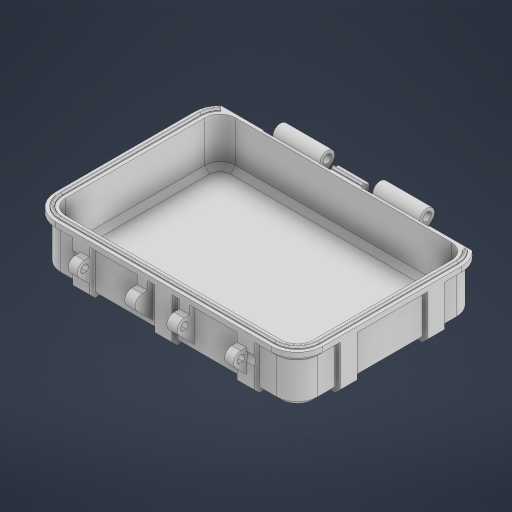
# Autodesk Inventor part: universal_box-lid
Saved by Autodesk Inventor 2024 (Build 280153000, 153)
## iProperties
Created: 2024-03-05
Part Number: universal_box-lid
Material: Všeobecné
Document SubType Name: Modeling
Designer: Simak
Density: 1 g/cm^3
Appearance: Výchozí
Author: Simak
Autodesk Inventor part; units mm, degrees
ref_plane "YZ Plane" through (0, 0, 0) normal (1, 0, 0) x (0, 1, 0)
ref_plane "XZ Plane" through (0, 0, 0) normal (0, 1, 0) x (-1, 0, 0)
ref_plane "XY Plane" through (0, 0, 0) normal (0, 0, 1) x (1, 0, 0)
sketch "velikost" plane through (0, 0, 0) normal (0, 1, 0) x (-1, 0, 0)
  line L0 (50, -35) -> (-50, -35)
  line L1 (-50, -35) -> (-50, 35)
  line L2 (-50, 35) -> (50, 35)
  line L3 (50, 35) -> (50, -35)
  line L4 (50, -35) -> (0, 0) construction
  line L5 (0, 0) -> (-50, -35) construction
  line L6 (0, 0) -> (-50, 35) construction
  dimension "d0" = 100
  dimension "d1" = 70
  constraints: 14 end point, 2 equal length, 2 parallel, 1 horizontal, 1 perpendicular
  measures "d0" distance of L0.start L0.end
  measures "d1" distance of L0.end L1.end
extrude "vyska" add sketch "velikost" along normal blind 20
fillet "Zaobleni_rohu" radius 8 4 edges at (-50, 10, 35) (50, 10, 35) (50, 10, -35) (-50, 10, -35)
shell "tloustka_sten" thickness 2 removed faces 1 at (-14, 20, 11.6667)
sketch "vyztuhy-velikost" plane through (0, 20, 0) normal (0, 1, 0) x (1, 0, 0)
  arc A0 (-42, 33) -> (-48, 27) centre (-42, 27) ccw projected
  line L0 (-42, 33) -> (42, 33) projected
  arc A1 (48, 27) -> (42, 33) centre (42, 27) ccw projected
  line L1 (48, 27) -> (48, -27) projected
  arc A2 (42, -33) -> (48, -27) centre (42, -27) ccw projected
  line L2 (42, -33) -> (-42, -33) projected
  arc A3 (-48, -27) -> (-42, -33) centre (-42, -27) ccw projected
  line L3 (-48, -27) -> (-48, 27) projected
  arc A4 (-42, 35) -> (-50, 27) centre (-42, 27) ccw projected
  line L4 (-50, 27) -> (-50, -27) projected
  arc A5 (-50, -27) -> (-42, -35) centre (-42, -27) ccw projected
  line L5 (-42, -35) -> (42, -35) projected
  arc A6 (42, -35) -> (50, -27) centre (42, -27) ccw projected
  line L6 (50, -27) -> (50, 27) projected
  arc A7 (50, 27) -> (42, 35) centre (42, 27) ccw projected
  line L7 (42, 35) -> (-42, 35) projected
  line L8 (-35.3333, 35) -> (-35.3333, 37)
  line L9 (-35.3333, 37) -> (-28.6667, 37)
  line L10 (-28.6667, 37) -> (-28.6667, 35)
  line L11 (-3.3333, 35) -> (-3.3333, 37)
  line L12 (-3.3333, 37) -> (3.3333, 37)
  line L13 (3.3333, 37) -> (3.3333, 35)
  line L14 (28.6667, 35) -> (28.6667, 37)
  line L15 (28.6667, 37) -> (35.3333, 37)
  line L16 (35.3333, 37) -> (35.3333, 35)
  line L17 (42, 35) -> (-42, 35) projected
  line L18 (-3.3333, 37) -> (0, 35) construction
  line L19 (3.3333, 37) -> (0, 35) construction
  line L20 (-28.6667, 37) -> (-3.3333, 37) construction
  line L21 (3.3333, 37) -> (28.6667, 37) construction
  line L22 (-35.3333, 37) -> (-42, 37) construction
  line L23 (-42, 37) -> (-42, 35) construction
  line L24 (-48, 0) -> (48, 0)
  line L25 (0, 33) -> (0, -33)
  line L26 (42, -33) -> (-42, -33) projected
  line L27 (-50, -20.3333) -> (-52, -20.3333)
  line L28 (-52, -20.3333) -> (-52, -13.6667)
  line L29 (-52, -13.6667) -> (-50, -13.6667)
  line L30 (-50, 13.6667) -> (-52, 13.6667)
  line L31 (-52, 13.6667) -> (-52, 20.3333)
  line L32 (-52, 20.3333) -> (-50, 20.3333)
  line L33 (-52, -13.6667) -> (-52, 13.6667) construction
  line L34 (-52, -20.3333) -> (-52, -27) construction
  line L35 (-52, -27) -> (-50, -27) construction
  line L36 (-50, 27) -> (-50, -27) projected
  line L37 (-52, 20.3333) -> (-52, 27) construction
  line L38 (-52, 27) -> (-50, 27) construction
  line L39 (-50, 0) -> (-52, 13.6667) construction
  line L40 (-50, 0) -> (-52, -13.6667) construction
  line L41 (-35.3333, -35) -> (-35.3333, -37)
  line L42 (-35.3333, -37) -> (-28.6667, -37)
  line L43 (-28.6667, -37) -> (-28.6667, -35)
  line L44 (-3.3333, -35) -> (-3.3333, -37)
  line L45 (-3.3333, -37) -> (3.3333, -37)
  line L46 (3.3333, -37) -> (3.3333, -35)
  line L47 (28.6667, -35) -> (28.6667, -37)
  line L48 (28.6667, -37) -> (35.3333, -37)
  line L49 (35.3333, -37) -> (35.3333, -35)
  line L50 (42, -35) -> (-42, -35)
  line L51 (-3.3333, -37) -> (0, -35) construction
  line L52 (3.3333, -37) -> (0, -35) construction
  line L53 (-28.6667, -37) -> (-3.3333, -37) construction
  line L54 (3.3333, -37) -> (28.6667, -37) construction
  line L55 (-35.3333, -37) -> (-42, -37) construction
  line L56 (-42, -37) -> (-42, -35) construction
  line L57 (50, 27) -> (50, -27)
  line L58 (52, -13.6667) -> (52, 13.6667) construction
  line L59 (50, -20.3333) -> (52, -20.3333)
  line L60 (52, -20.3333) -> (52, -27) construction
  line L61 (52, -13.6667) -> (50, -13.6667)
  line L62 (52, -27) -> (50, -27) construction
  line L63 (52, -20.3333) -> (52, -13.6667)
  line L64 (52, 13.6667) -> (52, 20.3333)
  line L65 (52, 20.3333) -> (50, 20.3333)
  line L66 (50, 13.6667) -> (52, 13.6667)
  line L67 (50, 27) -> (50, -27)
  line L68 (52, 20.3333) -> (52, 27) construction
  line L69 (52, 27) -> (50, 27) construction
  line L70 (50, 0) -> (52, 13.6667) construction
  line L71 (50, 0) -> (52, -13.6667) construction
  point P0 (0, 0)
  point P1 (50, 20.3333)
  point P2 (50, 13.6667)
  point P3 (50, -13.6667)
  point P4 (50, -20.3333)
  point P5 (35.3333, -35)
  point P6 (28.6667, -35)
  point P7 (3.3333, -35)
  point P8 (-3.3333, -35)
  point P9 (-28.6667, -35)
  point P10 (-35.3333, -35)
  point P11 (-50, 20.3333)
  dimension "d6" = 2
  dimension "d7" = 6.6667
  dimension "d8" = 2
  constraints: 120 end point, 25 symmetric about line, 20 point on line, 14 equal length, 11 perpendicular, 5 midpoint, 5 vertical, 2 horizontal, 5 other
  measures "d6" distance of L9.end L10.end
  measures "d7" distance of L11.end L12.end
  measures "d8" distance of L33.start L29.end
extrude "vyztuhy" add sketch "vyztuhy-velikost" against normal up to surface (20 mm away) contours L8 L9 L10 L7 | L4 L30 L31 L32 | L11 L12 L13 L7 | L4 L27 L28 L29 | L14 L15 L16 L7 | L5 L43 L42 L41 | L65 L64 L66 L6 | L5 L46 L45 L44 | L61 L63 L59 L6 | L5 L49 L48 L47
chamfer "Zkoseni_spodku" distance 2 angle 45 36 edges at (-16, 0, 35) (16, 0, 35) (0, 0, 37) (32, 0, 37) (38.6667, 0, 35) (47.6569, 0, 32.6569) (50, 0, 23.6667) (52, 0, 17) (50, 0, 0) (52, 0, -17) (47.6569, 0, -32.6569) (38.6667, 0, -35) (50, 0, -23.6667) (32, 0, -37) (16, 0, -35) (0, 0, -37) (-16, 0, -35) (-32, 0, -37) (-38.6667, 0, -35) (-47.6569, 0, -32.6569) (-50, 0, -23.6667) (-52, 0, -17) (-50, 0, 0) (-52, 0, 17) (-50, 0, 23.6667) (-47.6569, 0, 32.6569) (-38.6667, 0, 35) (-32, 0, 37) (-48, 2, 0) (-46.2426, 2, 31.2426) (0, 2, 33) (46.2426, 2, 31.2426) (48, 2, 0) (46.2426, 2, -31.2426) (0, 2, -33) (-46.2426, 2, -31.2426)
sketch "Náčrt4" plane through (35.3333, 20, -35) normal (1, 0, 0) x (0, 0, -1)
  line L0 (-2, 0) -> (-2, -16) projected
  line L1 (2, 0) -> (2, -18) projected
  line L2 (-8, 0) -> (0, 0) projected
  line L3 (-0.7, 0) -> (-0.7, 0.3)
  line L4 (-0.7, 0.3) -> (0.7, 0.3)
  line L5 (0.7, 0.3) -> (0.7, 0)
  line L6 (-0.7, 0.3) -> (-2, 0.3) construction
  line L7 (0.7, 0.3) -> (2, 0.3) construction
  line L8 (2, 0) -> (0, 0) projected
  line L9 (2, -4) -> (-2, -4)
  line L10 (-0.6, 0.3) -> (-0.1631, 0.9157)
  arc A0 (0.1631, 0.9157) -> (-0.1631, 0.9157) centre (0, 0.8) ccw
  line L11 (0.1631, 0.9157) -> (0.6, 0.3)
  point P0 (-35, -20)
  point P1 (0, 0.3)
  point P2 (0, 1)
  dimension "d16" = 1.4
  dimension "d71" = 4
  dimension "d72" = 0.3
  dimension "d75" = 1
  dimension "d76" = 0.2
  dimension "d77" = 0.6
  constraints: 16 end point, 9 point on line, 5 perpendicular, 3 point on circle, 3 vertical alignment, 2 equal length, 2 tangent, 1 centre point, 1 midpoint
  measures "d16" distance of L3.end L4.end
  measures "d71" distance between parallel lines of L9 L8
  measures "d72" distance between parallel lines of L8 L4
  measures "d75" distance from line of L8 point (0, 1)
  measures "d76" radius of A0
  measures "d77" horizontal distance of L11.end A0.centre
sketch "Náčrt3" plane through (0, 20, 0) normal (0, 1, 0) x (1, 0, 0)
  arc A0 (-42, 33) -> (-48, 27) centre (-42, 27) ccw projected
  line L0 (-42, 33) -> (42, 33) projected
  arc A1 (48, 27) -> (42, 33) centre (42, 27) ccw projected
  line L1 (48, 27) -> (48, -27) projected
  arc A2 (42, -33) -> (48, -27) centre (42, -27) ccw projected
  line L2 (42, -33) -> (-42, -33) projected
  arc A3 (-48, -27) -> (-42, -33) centre (-42, -27) ccw projected
  line L3 (-48, -27) -> (-48, 27) projected
  arc A4 (-42, 35) -> (-50, 27) centre (-42, 27) ccw projected
  line L4 (-50, 27) -> (-50, 20.3333) projected
  line L5 (-52, 13.6667) -> (-50, 13.6667) projected
  line L6 (-50, 13.6667) -> (-50, -13.6667) projected
  line L7 (-50, -13.6667) -> (-52, -13.6667) projected
  line L8 (-52, -13.6667) -> (-52, -20.3333) projected
  arc A5 (-50, -27) -> (-42, -35) centre (-42, -27) ccw projected
  line L9 (-42, -35) -> (-35.3333, -35) projected
  line L10 (-35.3333, -35) -> (-35.3333, -37) projected
  line L11 (-35.3333, -37) -> (-28.6667, -37) projected
  line L12 (-28.6667, -37) -> (-28.6667, -35) projected
  line L13 (-28.6667, -35) -> (-3.3333, -35) projected
  line L14 (-3.3333, -35) -> (-3.3333, -37) projected
  line L15 (-3.3333, -37) -> (3.3333, -37) projected
  line L16 (3.3333, -37) -> (3.3333, -35) projected
  line L17 (3.3333, -35) -> (28.6667, -35) projected
  line L18 (28.6667, -35) -> (28.6667, -37) projected
  line L19 (28.6667, -37) -> (35.3333, -37) projected
  line L20 (35.3333, -37) -> (35.3333, -35) projected
  line L21 (35.3333, -35) -> (42, -35) projected
  arc A6 (42, -35) -> (50, -27) centre (42, -27) ccw projected
  line L22 (50, -27) -> (50, -20.3333) projected
  line L23 (52, -13.6667) -> (50, -13.6667) projected
  line L24 (50, -13.6667) -> (50, 13.6667) projected
  line L25 (50, 13.6667) -> (52, 13.6667) projected
  line L26 (52, 13.6667) -> (52, 20.3333) projected
  arc A7 (50, 27) -> (42, 35) centre (42, 27) ccw projected
  line L27 (42, 35) -> (35.3333, 35) projected
  line L28 (35.3333, 35) -> (35.3333, 37) projected
  line L29 (35.3333, 37) -> (28.6667, 37) projected
  line L30 (28.6667, 37) -> (28.6667, 35) projected
  line L31 (28.6667, 35) -> (3.3333, 35) projected
  line L32 (3.3333, 35) -> (3.3333, 37) projected
  line L33 (3.3333, 37) -> (-3.3333, 37) projected
  line L34 (-3.3333, 37) -> (-3.3333, 35) projected
  line L35 (-3.3333, 35) -> (-28.6667, 35) projected
  line L36 (-28.6667, 35) -> (-28.6667, 37) projected
  line L37 (-28.6667, 37) -> (-35.3333, 37) projected
  line L38 (-35.3333, 37) -> (-35.3333, 35) projected
  line L39 (-35.3333, 35) -> (-42, 35) projected
  line L40 (-50, 20.3333) -> (-52, 20.3333) projected
  line L41 (-52, 20.3333) -> (-52, 13.6667) projected
  line L42 (-52, -20.3333) -> (-50, -20.3333) projected
  line L43 (-50, -20.3333) -> (-50, -27) projected
  line L44 (50, -20.3333) -> (52, -20.3333) projected
  line L45 (52, -20.3333) -> (52, -13.6667) projected
  line L46 (52, 20.3333) -> (50, 20.3333) projected
  line L47 (50, 20.3333) -> (50, 27) projected
  point P0 (0, 0)
sweep "tesnici_drazka" add profiles "Náčrt4" path "Náčrt3" path curves L0 A0 L3 A3 L2 A2 L1 A1
chamfer "tesnici_drazka-zkoseni" distance 2 angle 45 18 edges at (49.0711, 16, -34.0711) (38.6667, 16, -37) (52, 16, -23.6667) (16, 16, -37) (-16, 16, -37) (52, 16, 0) (52, 16, 23.6667) (49.0711, 16, 34.0711) (38.6667, 16, 37) (-49.0711, 16, -34.0711) (-52, 16, -23.6667) (-38.6667, 16, -37) (-52, 16, 0) (-49.0711, 16, 34.0711) (-38.6667, 16, 37) (-52, 16, 23.6667) (16, 16, 37) (-16, 16, 37)
sketch "Náčrt16" plane through (28.6667, 0, -35) normal (-1, 0, 0) x (0, 0, 1)
  line L0 (-2, 18) -> (-2, 2) projected
  line L1 (0, 0) -> (-2, 2) projected
  line L2 (2, 0) -> (0, 0) projected
  line L3 (0, 2) -> (2, 0) projected
  line L4 (0, 16) -> (0, 2) projected
  line L5 (-2, 18) -> (0, 16) projected
  line L6 (8, 20) -> (-2, 20) projected
  circle A0 centre (-2, 20) radius 1.65
  circle A1 centre (-2, 20) radius 2.7
  circle A2 centre (-2, 20) radius 2.875
  circle A3 centre (-2, 20) radius 3.025
  line L7 (0, 13.9341) -> (-4.0329, 17.9671)
  point P0 (35, 0)
  point P1 (0.875, 20)
  point P2 (-1.1092, 17.1092)
  point P3 (1.025, 20)
  point P4 (-3.3677, 17.3019)
  point P5 (-2, 15.9341)
  point P6 (-2, 16.975)
  dimension "d148" = 5.75
  dimension "d147" = 3.3
  dimension "d149" = 5.4
  dimension "d150" = 0.15
  dimension "d151" = 45
  constraints: 3 centre point, 3 coincident, 2 end point, 1 point on line, 4 other
  measures "d147" diameter of A0
  measures "d149" diameter of A1
  measures "d151" angle of L4 L7
extrude "Vysunutí23" cut sketch "Náčrt16" along normal blind 22.65 and the other way blind 3.65 contours L5 A1 L0 | L0 A1 L5 | A1 L5 A2 L0 | L0 A2 L6 A1 | A1 L6 A2 L5 | A2 L5 A3 L0 | L0 A3 L7 A2 | A2 L6 A3 L5 | L7 A3 L6 A2 | A0
extrude "Vysunutí24" cut sketch "Náčrt16" against normal through all contours L5 A1 L0 | L0 A1 L5 | A0
extrude "Vysunutí25" add sketch "Náčrt16" along normal blind 18.4 contours L5 A1 L0 | L0 A1 L5 | A1 L5 A2 L0 | L0 A2 L6 A1 | A1 L6 A2 L5 | A2 L5 A3 L0 | L0 A3 L7 A2 | A2 L6 A3 L5 | A3 L5 L4 L7 L0 | L0 L7 A3
extrude "Vysunutí26" cut sketch "Náčrt16" along normal blind 0.1 contours L5 A1 L0 | L0 A1 L5 | A1 L5 A2 L0 | L0 A2 L6 A1 | A1 L6 A2 L5 | A2 L5 A3 L0 | L0 A3 L7 A2 | A2 L6 A3 L5 | L0 L7 A3 | L7 A3 L6 A2 | A0
sketch "Náčrt17" plane through (0, 20, 0) normal (0, 1, 0) x (1, 0, 0)
  arc A0 (-42, 33) -> (-48, 27) centre (-42, 27) ccw projected
  line L0 (-42, 33) -> (42, 33) projected
  arc A1 (48, 27) -> (42, 33) centre (42, 27) ccw projected
  line L1 (48, 27) -> (48, -27) projected
  arc A2 (42, -33) -> (48, -27) centre (42, -27) ccw projected
  line L2 (42, -33) -> (-42, -33) projected
  arc A3 (-48, -27) -> (-42, -33) centre (-42, -27) ccw projected
  line L3 (-48, -27) -> (-48, 27) projected
  arc A4 (-42, 34.3) -> (-49.3, 27) centre (-42, 27) ccw projected
  line L4 (-49.3, 27) -> (-49.3, -27) projected
  arc A5 (-49.3, -27) -> (-42, -34.3) centre (-42, -27) ccw projected
  line L5 (-42, -34.3) -> (42, -34.3) projected
  arc A6 (42, -34.3) -> (49.3, -27) centre (42, -27) ccw projected
  line L6 (49.3, -27) -> (49.3, 27) projected
  arc A7 (49.3, 27) -> (42, 34.3) centre (42, 27) ccw projected
  line L7 (42, 34.3) -> (32.3167, 34.3) projected
  line L8 (32.3167, 34.3) -> (32.3167, 33.975) projected
  line L9 (32.3167, 33.975) -> (28.5667, 33.975) projected
  line L10 (28.5667, 33.975) -> (28.5667, 34.125) projected
  line L11 (28.5667, 34.125) -> (10.2667, 34.125) projected
  line L12 (10.2667, 33.975) -> (10.2667, 34.125) projected
  line L13 (10.2667, 33.975) -> (6.0167, 33.975) projected
  line L14 (6.0167, 33.975) -> (6.0167, 34.3) projected
  line L15 (6.0167, 34.3) -> (-42, 34.3) projected
  arc A8 (-42, 37) -> (-52, 27) centre (-42, 27) ccw projected
  line L16 (-52, 27) -> (-52, -27) projected
  arc A9 (-52, -27) -> (-42, -37) centre (-42, -27) ccw projected
  line L17 (-42, -37) -> (42, -37) projected
  arc A10 (42, -37) -> (52, -27) centre (42, -27) ccw projected
  line L18 (52, -27) -> (52, 27) projected
  arc A11 (52, 27) -> (48.8345, 34.3) centre (42, 27) ccw projected
  line L19 (48.8345, 34.3) -> (46.7329, 34.3) projected
  arc A12 (50.7, 27) -> (46.7329, 34.3) centre (42, 27) ccw projected
  line L20 (50.7, -27) -> (50.7, 27) projected
  arc A13 (42, -35.7) -> (50.7, -27) centre (42, -27) ccw projected
  line L21 (-42, -35.7) -> (42, -35.7) projected
  arc A14 (-50.7, -27) -> (-42, -35.7) centre (-42, -27) ccw projected
  line L22 (-50.7, 27) -> (-50.7, -27) projected
  arc A15 (-42, 35.7) -> (-50.7, 27) centre (-42, 27) ccw projected
  spline S0 degree 8 poles (42, 36.3737) (42.5163, 36.3737) (43.0323, 36.3475) (43.5473, 36.2951) (44.0603, 36.2176) (44.5703, 36.1177) (45.0764, 35.9985) (45.5774, 35.8641) (46.2861, 35.6565) (46.4987, 35.592) (46.71, 35.5258) (46.9199, 35.4585) (47.1283, 35.3905) (47.3351, 35.3221) (47.5401, 35.2539) (47.7432, 35.1863) knots 0 0 0 0 0 0 0 0 0 0.698385 0.698385 0.698385 0.698385 0.698385 0.698385 0.698385 1 1 1 1 1 1 1 1 1 projected
  line L23 (35.3333, 36.3737) -> (42, 36.3737) projected
  line L24 (35.3333, 37) -> (35.3333, 36.3737) projected
  line L25 (32.3167, 37) -> (35.3333, 37) projected
  line L26 (32.3167, 34.3) -> (32.3167, 37) projected
  line L27 (42, 34.3) -> (32.3167, 34.3) projected
  line L28 (32.3167, 34.3167) -> (32.3167, 34.3) projected
  line L29 (43.1071, 34.3167) -> (32.3167, 34.3167) projected
  line L30 (46.707, 34.3167) -> (46.5195, 34.3167) projected
  line L31 (48.8345, 34.3) -> (46.7329, 34.3) projected
  spline S1 degree 6 poles (47.7432, 35.1863) (47.8272, 35.1273) (47.9089, 35.0685) (47.9878, 35.0102) (48.0637, 34.9527) (48.1363, 34.8964) (48.2493, 34.807) (48.2917, 34.773) (48.3326, 34.7397) (48.3719, 34.7073) (48.4096, 34.6759) (48.4724, 34.6229) (48.4985, 34.6008) (48.5235, 34.5793) (48.5475, 34.5586) (48.5703, 34.5387) (48.6714, 34.4501) (48.7361, 34.3916) (48.7852, 34.3462) (48.818, 34.3154) (48.8345, 34.3) (48.8345, 34.3) knots 0 0 0 0 0 0 0 0.258993 0.258993 0.258993 0.258993 0.258993 0.423699 0.423699 0.423699 0.423699 0.423699 0.547895 0.547895 0.547895 0.547895 0.547895 1 1 1 1 1 1 1 projected
  line L32 (32.3167, 33.975) -> (32.3167, 33)
  line L33 (42, 27) -> (48, 33.3)
  line L34 (6.0167, 35.7) -> (-42, 35.7) projected
  line L35 (6.0167, 35.7) -> (6.0167, 37) projected
  line L36 (6.0167, 37) -> (-42, 37) projected
  point P0 (0, 0)
  point P1 (47.0345, 32.2862)
  point P2 (46.7329, 24.3)
  point P3 (46.7329, 34.3)
  point P4 (51.7329, 54.3)
  dimension "d162" = 1
  constraints: 4 end point, 1 horizontal alignment, 1 perpendicular, 1 point on circle, 1 point on line, 5 other
  measures "d162" distance from line of L19 L33.end
extrude "Vysunutí27" cut sketch "Náčrt17" along normal through all contours L26 L25 L24 L23 S0 S1 L19 A12 L33 A7 L7
sketch "Náčrt18" plane through (28.5667, 0, -35) normal (1, 0, 0) x (0, 0, -1)
  line L0 (4.0329, 17.9671) -> (2, 15.9341) projected
  arc A0 (4.0329, 17.9671) -> (-0.875, 20) centre (2, 20) ccw projected
  line L1 (-1.025, 20) -> (-0.875, 20) projected
  arc A1 (-1.025, 20) -> (2, 16.975) centre (2, 20) ccw projected
  line L2 (2, 15.9341) -> (2, 16.975) projected
  circle A2 centre (2, 20) radius 1.65 projected
  circle A3 centre (2, 20) radius 2.875
  line L3 (-0.139, 17.861) -> (2, 15.722)
  line L4 (2, 18) -> (2, 2) projected
  arc A4 (-1.025, 20) -> (1.1092, 17.1092) centre (2, 20) ccw projected
  point P0 (-35, 0)
  point P1 (-0.139, 17.861)
  dimension "d165" = 45
  constraints: 3 point on circle, 2 end point, 1 coincident, 1 horizontal alignment, 1 point on line, 1 tangent, 2 other
  measures "d165" angle of L4 L3
extrude "Vysunutí28" cut sketch "Náčrt18" along normal up to surface (3.75 mm away) contours L4 L3 A1 L2
sketch "Náčrt19" plane through (10.2667, 0, -35) normal (-1, 0, 0) x (0, 0, 1)
  line L0 (-4.0329, 17.9671) -> (-1.8939, 15.8281) projected
  arc A0 (0.875, 20) -> (-4.0329, 17.9671) centre (-2, 20) ccw projected
  line L1 (1.025, 20) -> (0.875, 20) projected
  arc A1 (0.139, 17.861) -> (1.025, 20) centre (-2, 20) ccw projected
  line L2 (0.139, 17.861) -> (-1.8939, 15.8281) projected
  circle A2 centre (-2, 20) radius 1.65 projected
  point P0 (35, 0)
extrude "Vysunutí29" cut sketch "Náčrt19" along normal up to surface (4.25 mm away)
mirror "Zrcadlit4" about plane through (0, 0, 0) normal (1, 0, 0) of "Vysunutí23", "Vysunutí24", "Vysunutí25", "Vysunutí26", "Vysunutí27", "Vysunutí28", "Vysunutí29"
sketch "latch-main_nacrt" plane through (28.6667, 0, 33) normal (-1, 0, 0) x (0, 0, 1)
  line L0 (4, 18) -> (4, 2) projected
  line L1 (2, 0) -> (4, 2) projected
  line L2 (0, 0) -> (2, 0) projected
  line L3 (2, 2) -> (0, 0) projected
  line L4 (2, 16) -> (2, 2) projected
  line L5 (4, 18) -> (2, 16) projected
  line L6 (4, 20) -> (-6, 20) projected
  line L7 (2.7, 20.3) -> (-6, 20.3) projected
  line L8 (1.25, 23) -> (1.25, 25) projected
  line L9 (2.7, 20.3) -> (2.7, 20) projected
  line L10 (4, 20) -> (4, 18) projected
  circle A0 centre (6.05, 11.8) radius 1.55
  line L11 (5.3, 10.4435) -> (5.3, 10.6)
  line L12 (5.3, 10.6) -> (6.8, 10.6)
  line L13 (6.8, 10.6) -> (6.8, 10.4435)
  circle A1 centre (6.05, 11.8) radius 2.875
  line L14 (6.05, 14.675) -> (2, 14.675)
  line L15 (2, 3.6841) -> (8.0829, 9.7671)
  circle A2 centre (6.05, 11.8) radius 2.7
  point P0 (-33, 0)
  point P1 (-6, 20.3)
  point P2 (4, 13.8157)
  point P3 (4, 9.7843)
  dimension "d52" = 3.1
  dimension "d53" = 8.2
  dimension "d54" = 4.05
  dimension "d55" = 2.75
  dimension "d56" = 1.5
  dimension "d57" = 5.75
  dimension "d58" = 45
  dimension "d63" = 5.4
  constraints: 10 end point, 4 point on circle, 3 centre point, 3 perpendicular, 2 coincident, 2 point on line, 2 tangent, 1 parallel, 1 vertical, 2 other
  measures "d52" diameter of A0
  measures "d54" distance from line of L4 A0.centre
  measures "d56" distance of L11.end L12.end
  measures "d57" diameter of A1
  measures "d58" angle of L4 L15
  measures "d63" diameter of A2
extrude "Vysunutí14" cut sketch "latch-main_nacrt" against normal up to next contours A2 L0 | L0 A2
extrude "Vysunutí12" add sketch "latch-main_nacrt" against normal blind 3.5 contours L14 A1 L0 | L0 A1 L15 L4 L14 | A1 L0 A2 | L0 A2 A1 | A2 L0 | L0 A2 | A1 L15 L0 | L11 L12 L13 A0 picked at (5.9979, 10.486)
ref_plane "Pracovní rovina3" through (10.1667, 0, 33) normal (-1, 0, 0) x (0, 0, 1)
sketch "Náčrt10" plane through (10.1667, 0, 33) normal (-1, 0, 0) x (0, 0, 1)
  arc A0 (6.8, 10.4435) -> (5.3, 10.4435) centre (6.05, 11.8) ccw projected
  line L0 (6.8, 10.4435) -> (6.8, 10.6) projected
  line L1 (6.8, 10.6) -> (5.3, 10.6) projected
  line L2 (5.3, 10.6) -> (5.3, 10.4435) projected
  line L3 (4, 5.6841) -> (8.0829, 9.7671) projected
  arc A1 (8.0829, 9.7671) -> (6.05, 14.675) centre (6.05, 11.8) ccw projected
  line L4 (6.05, 14.675) -> (4, 14.675) projected
  line L5 (4, 18) -> (4, 14.675) projected
  line L6 (2, 16) -> (4, 18) projected
  line L7 (2, 2) -> (2, 16) projected
  line L8 (0, 0) -> (2, 2) projected
  line L9 (2, 0) -> (0, 0) projected
  line L10 (4, 2) -> (2, 0) projected
  line L11 (4, 5.6841) -> (4, 2) projected
  line L12 (4, 14.675) -> (2, 14.675)
  line L13 (4, 5.6841) -> (2, 3.6841)
  line L14 (4, 14.675) -> (2, 16)
  point P0 (-33, 0)
  constraints: 6 end point, 2 collinear, 2 point on line
extrude "Vysunutí15" add sketch "Náčrt10" along normal blind 4 contours L13 L7 L12 L4 A1 L3 | L7 L14 L12 | L14 L6 L5
sketch "Náčrt12" plane through (6.1667, 0, 33) normal (-1, 0, 0) x (0, 0, 1)
  line L0 (2, 3.6841) -> (8.0829, 9.7671) projected
  arc A0 (8.0829, 9.7671) -> (6.05, 14.675) centre (6.05, 11.8) ccw projected
  line L1 (6.05, 14.675) -> (4, 14.675) projected
  line L2 (6.8, 10.6) -> (5.3, 10.6) projected
  line L3 (5.3, 10.6) -> (5.3, 10.4435) projected
  arc A1 (6.8, 10.4435) -> (5.3, 10.4435) centre (6.05, 11.8) ccw projected
  line L4 (6.8, 10.4435) -> (6.8, 10.6) projected
  line L5 (4, 14.675) -> (4, 18) projected
  line L6 (2, 16) -> (4, 18) projected
  line L7 (2, 3.6841) -> (2, 16) projected
  point P0 (-33, 0)
extrude "Vysunutí16" add sketch "Náčrt12" against normal blind 0.5 contours L2 L3 A1 L4
mirror "latch-zrcadleni" about plane through (0, 0, 0) normal (1, 0, 0) of "Vysunutí16", "Vysunutí14", "Vysunutí12", "Vysunutí15"
fillet "Zaoblení2" radius 1 8 edges at (-38.6667, 17.3736, -36.3737) (-44.9352, 17.4845, -36.019) (-48.5393, 18.8323, -34.5656) (-33.825, 17.3, -37) (33.825, 17.3, -37) (44.9352, 17.4845, -36.019) (38.6667, 17.3736, -36.3737) (48.5393, 18.8323, -34.5656)
ref_plane "Pracovní rovina4" through (-10.1667, 0, 33) normal (-1, 0, 0) x (0, 0, 1)
